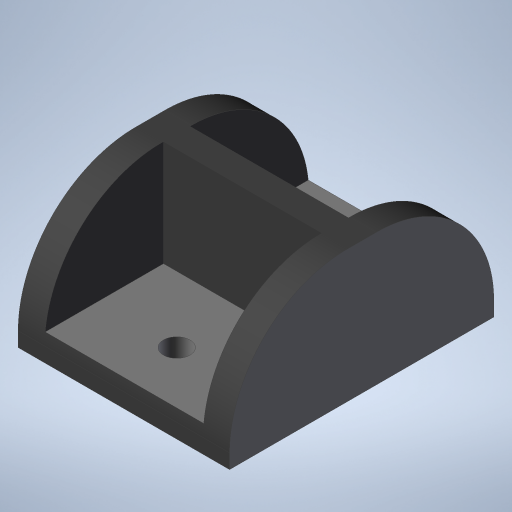
# Autodesk Inventor part: LightSensor01
Saved by Autodesk Inventor 2023 (Build 270158000, 158)
## iProperties
Created: 2023-03-20
Part Number: LightSensor01
Material: Generic
Document SubType Name: Modeling
Designer: ringl
Density: 1 g/cm^3
Appearance: Default
Author: ringl
Autodesk Inventor part; units mm, degrees
ref_plane "YZ Plane" through (0, 0, 0) normal (1, 0, 0) x (0, 1, 0)
ref_plane "XZ Plane" through (0, 0, 0) normal (0, 1, 0) x (-1, 0, 0)
ref_plane "XY Plane" through (0, 0, 0) normal (0, 0, 1) x (1, 0, 0)
sketch "Sketch1" plane through (0, 0, 0) normal (0, 1, 0) x (-1, 0, 0)
  line L0 (0, 0) -> (40, 0)
  line L1 (40, 0) -> (40, -50)
  line L2 (40, -50) -> (0, -50)
  line L3 (0, -50) -> (0, 0)
  circle A0 centre (20, -10) radius 2.5
  circle A1 centre (20, -40) radius 2.5
  dimension "d0" = 40
  dimension "d1" = 50
  dimension "d2" = 5
  dimension "d3" = 5
  dimension "d4" = 10
  dimension "d5" = 10
  dimension "d6" = 20
  constraints: 8 end point, 2 centre point, 2 parallel, 1 horizontal, 1 perpendicular, 1 vertical alignment
  measures "d0" distance of L1.end L2.end
  measures "d1" distance of L0.end L1.end
  measures "d2" diameter of A0
  measures "d3" diameter of A1
  measures "d4" distance from line of L0 A0.centre
  measures "d5" distance from line of L2 A1.centre
  measures "d6" distance from line of L3 A1.centre
extrude "Extrusion1" add sketch "Sketch1" along normal blind 5
sketch "Sketch2" plane through (0, 5, 0) normal (0, 1, 0) x (1, 0, 0)
  line L0 (-40, 50) -> (-40, 0) projected
  line L1 (0, 0) -> (0, 50) projected
  line L2 (-40, 22.5) -> (0, 22.5)
  line L3 (0, 22.5) -> (0, 27.5)
  line L4 (0, 27.5) -> (-40, 27.5)
  line L5 (-40, 27.5) -> (-40, 22.5)
  line L6 (-40, 0) -> (0, 0) projected
  line L7 (0, 50) -> (-40, 50) projected
  line L8 (-40, 50) -> (-35, 50)
  line L9 (-35, 50) -> (-35, 0)
  line L10 (-35, 0) -> (-40, 0)
  line L11 (-40, 0) -> (-40, 50)
  line L12 (-5, 0) -> (0, 0)
  line L13 (0, 0) -> (0, 50)
  line L14 (0, 50) -> (-5, 50)
  line L15 (-5, 50) -> (-5, 0)
  point P0 (0, 22.5)
  point P1 (-5, 22.5)
  point P2 (-5, 27.5)
  point P3 (-35, 22.5)
  point P4 (-35, 27.5)
  dimension "d9" = 5
  dimension "d10" = 22.5
  dimension "d13" = 5
  dimension "d14" = 5
  constraints: 24 end point, 6 parallel, 4 point on line, 3 horizontal, 3 perpendicular
  measures "d9" distance between parallel lines of L2 L4
  measures "d10" distance between parallel lines of L6 L2
  measures "d13" distance between parallel lines of L0 L9
  measures "d14" distance between parallel lines of L1 L15
extrude "Extrusion2" add sketch "Sketch2" along normal blind 20 contours L7 L9 L4 L0 | L4 L9 L2 L0 | L2 L9 L6 L0 | L4 L15 L2 L9 | L7 L1 L4 L15 | L4 L1 L2 L15 | L2 L1 L6 L15
fillet "Fillet1" radius 22.25 4 edges at (-37.5, 25, 0) (-37.5, 25, -50) (-2.5, 25, -50) (-2.5, 25, 0)
body "Solid1"
